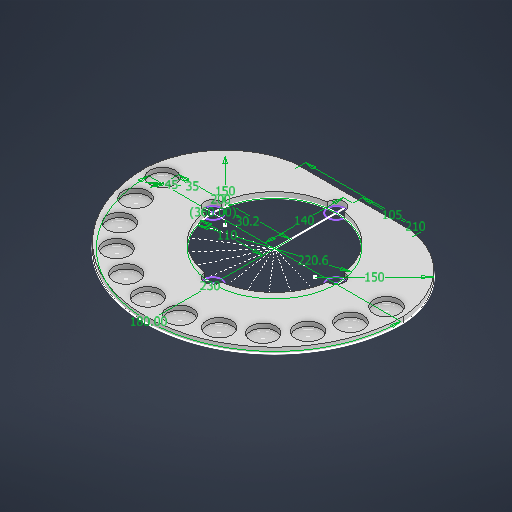
# Autodesk Inventor part: BasePlate
Saved by Autodesk Inventor 2026.2 (Build 302298000, 298)
## iProperties
Created: 2025-12-30
Part Number: BasePlate
Material: Generic
Document SubType Name: Modeling
Designer: Cobble
Density: 1 g/cm^3
Appearance: Default
Author: Cobble
Autodesk Inventor part; units mm, degrees
ref_plane "YZ Plane" through (0, 0, 0) normal (1, 0, 0) x (0, 1, 0)
ref_plane "XZ Plane" through (0, 0, 0) normal (0, 1, 0) x (-1, 0, 0)
ref_plane "XY Plane" through (0, 0, 0) normal (0, 0, 1) x (1, 0, 0)
sketch "Sketch1" plane through (0, 0, 0) normal (0, 0, 1) x (1, 0, 0)
  line L0 (0, 0) -> (-200, 0) construction
  circle A0 centre (-200, 0) radius 17.5
  circle A1 centre (-200, 0) radius 22.5
  line L1 (0, 0) -> (-191.898595, -56.346511) construction
  circle A2 centre (-191.898595, -56.346511) radius 17.5
  circle A3 centre (-191.898595, -56.346511) radius 22.5
  line L2 (0, 0) -> (-168.250707, -108.128163) construction
  circle A4 centre (-168.250707, -108.128163) radius 17.5
  circle A5 centre (-168.250707, -108.128163) radius 22.5
  line L3 (0, 0) -> (-130.972147, -151.149915) construction
  circle A6 centre (-130.972147, -151.149915) radius 17.5
  circle A7 centre (-130.972147, -151.149915) radius 22.5
  line L4 (0, 0) -> (-83.083003, -181.926399) construction
  circle A8 centre (-83.083003, -181.926399) radius 17.5
  circle A9 centre (-83.083003, -181.926399) radius 22.5
  line L5 (0, 0) -> (-28.462968, -197.964288) construction
  circle A10 centre (-28.462968, -197.964288) radius 17.5
  circle A11 centre (-28.462968, -197.964288) radius 22.5
  line L6 (0, 0) -> (28.462968, -197.964288) construction
  circle A12 centre (28.462968, -197.964288) radius 17.5
  circle A13 centre (28.462968, -197.964288) radius 22.5
  line L7 (0, 0) -> (83.083003, -181.926399) construction
  circle A14 centre (83.083003, -181.926399) radius 17.5
  circle A15 centre (83.083003, -181.926399) radius 22.5
  line L8 (0, 0) -> (130.972147, -151.149915) construction
  circle A16 centre (130.972147, -151.149915) radius 17.5
  circle A17 centre (130.972147, -151.149915) radius 22.5
  line L9 (0, 0) -> (168.250707, -108.128163) construction
  circle A18 centre (168.250707, -108.128163) radius 17.5
  circle A19 centre (168.250707, -108.128163) radius 22.5
  line L10 (0, 0) -> (191.898595, -56.346511) construction
  circle A20 centre (191.898595, -56.346511) radius 17.5
  circle A21 centre (191.898595, -56.346511) radius 22.5
  line L11 (0, 0) -> (200, 0) construction
  circle A22 centre (200, 0) radius 17.5
  circle A23 centre (200, 0) radius 22.5
  circle A24 centre (-200, 0) radius 0 construction
  circle A25 centre (200, 0) radius 0 construction
  arc A26 (-200, 0) -> (-200, 0) centre (-200, 0) ccw
  arc A27 (200, 0) -> (200, 0) centre (200, 0) ccw
  line L12 (0, 0) -> (-200, 0) construction
  circle A28 centre (0, 0) radius 110.3
  circle A29 centre (-110, 0) radius 15.1
  arc A30 (-230, 0) -> (230, 0) centre (0, 0) ccw
  line L13 (0, 0) -> (0, 140)
  line L14 (0, 140) -> (-105, 140)
  line L15 (0, 140) -> (105, 140)
  arc A31 (230, 0) -> (105, 140) centre (80.210153, -7.937363) ccw
  arc A32 (-105, 140) -> (-230, 0) centre (-80.210153, -7.937363) ccw
  circle A33 centre (0, -110) radius 15.1
  circle A34 centre (110, 0) radius 15.1
  circle A35 centre (0, 110) radius 15.1
  point P0 (-166.666667, 74.535599)
  point P1 (-109.264, -15.082052)
  point P2 (-109.264, 15.082052)
  point P3 (15.082052, 109.264)
  point P4 (109.264, 15.082052)
  point P5 (109.264, -15.082052)
  point P6 (15.082052, -109.264)
  point P7 (-15.082052, -109.264)
  point P8 (-15.082052, 109.264)
  dimension "d1" = 35
  dimension "d2" = 45
  dimension "d5" = 180
  dimension "d35" = 200
  dimension "d36" = 220.6
  dimension "d43" = 30.2
  dimension "d48" = 230
  dimension "d49" = 140
  dimension "d53" = 105
  dimension "d54" = 150
  dimension "d55" = 150
  dimension "d56" = 210
  dimension "d58" = 110
  dimension "d61" = 360
  constraints: 36 centre point, 32 end point, 31 coincident, 8 coincident with centre, 6 point on circle, 4 horizontal, 2 point on line, 1 perpendicular, 87 other
  measures "d1" diameter of A0
  measures "d2" diameter of A1
  measures "d35" distance of L0.start L0.end
  measures "d36" diameter of A28
  measures "d43" diameter of A29
  measures "d48" radius of A30
  measures "d49" distance of L13.start L13.end
  measures "d53" distance of L13.end L15.end
  measures "d54" radius of A31
  measures "d55" radius of A32
  measures "d56" distance of L15.end L14.end
  measures "d58" distance of L0.start A29.centre
sketch "Sketch1 outline for Extrusion1" plane through (0, 0, 0) normal (0, 0, 1) x (1, 0, 0)
  line L0 (0, 140) -> (-105, 140)
  line L1 (105, 140) -> (0, 140)
  arc A0 (-105, 140) -> (-230, 0) centre (-80.210153, -7.937363) ccw
  arc A1 (230, 0) -> (105, 140) centre (80.210153, -7.937363) ccw
  arc A2 (-230, 0) -> (230, 0) centre (0, 0) ccw
  circle A3 centre (-130.972147, -151.149915) radius 22.5
  circle A4 centre (-83.083003, -181.926399) radius 22.5
  circle A5 centre (-28.462968, -197.964288) radius 22.5
  circle A6 centre (-168.250707, -108.128163) radius 22.5
  circle A7 centre (-191.898595, -56.346511) radius 22.5
  circle A8 centre (28.462968, -197.964288) radius 22.5
  circle A9 centre (83.083003, -181.926399) radius 22.5
  circle A10 centre (130.972147, -151.149915) radius 22.5
  circle A11 centre (168.250707, -108.128163) radius 22.5
  circle A12 centre (191.898595, -56.346511) radius 22.5
  circle A13 centre (-200, 0) radius 22.5
  arc A14 (-15.082052, 109.264) -> (15.082052, 109.264) centre (0, 110) cw
  arc A15 (-109.264, 15.082052) -> (-15.082052, 109.264) centre (0, 0) cw
  arc A16 (-109.264, -15.082052) -> (-109.264, 15.082052) centre (-110, 0) cw
  arc A17 (-15.082052, -109.264) -> (-109.264, -15.082052) centre (0, 0) cw
  arc A18 (15.082052, -109.264) -> (-15.082052, -109.264) centre (0, -110) cw
  arc A19 (109.264, -15.082052) -> (15.082052, -109.264) centre (0, 0) cw
  arc A20 (109.264, 15.082052) -> (109.264, -15.082052) centre (110, 0) cw
  arc A21 (15.082052, 109.264) -> (109.264, 15.082052) centre (0, 0) cw
  circle A22 centre (200, 0) radius 22.5
extrude "Extrusion1" add sketch "Sketch1 outline for Extrusion1" along normal blind 10
sketch "Sketch1 outline for Extrusion2" plane through (0, 0, 0) normal (0, 0, 1) x (1, 0, 0)
  circle A0 centre (-200, 0) radius 22.5
  circle A1 centre (-191.898595, -56.346511) radius 22.5
  circle A2 centre (-168.250707, -108.128163) radius 22.5
  circle A3 centre (-130.972147, -151.149915) radius 22.5
  circle A4 centre (-83.083003, -181.926399) radius 22.5
  circle A5 centre (-28.462968, -197.964288) radius 22.5
  circle A6 centre (28.462968, -197.964288) radius 22.5
  circle A7 centre (83.083003, -181.926399) radius 22.5
  circle A8 centre (130.972147, -151.149915) radius 22.5
  circle A9 centre (168.250707, -108.128163) radius 22.5
  circle A10 centre (191.898595, -56.346511) radius 22.5
  circle A11 centre (200, 0) radius 22.5
extrude "Extrusion2" add sketch "Sketch1 outline for Extrusion2" along normal blind 2
body "Solid1"
